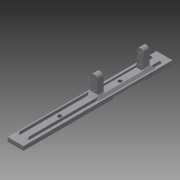
# Autodesk Inventor part: Top piece
Saved by Autodesk Inventor 2015 (Build 190159000, 159)
## iProperties
Created: 2014-11-22
Part Number: Top piece
Material: Generic
Document SubType Name: Modeling
Designer: jesse
Density: 1 g/cm^3
Appearance: Default
Author: jesse
Autodesk Inventor part; units mm, degrees
ref_plane "YZ Plane" through (0, 0, 0) normal (1, 0, 0) x (0, 1, 0)
ref_plane "XZ Plane" through (0, 0, 0) normal (0, 1, 0) x (-1, 0, 0)
ref_plane "XY Plane" through (0, 0, 0) normal (0, 0, 1) x (1, 0, 0)
sketch "Sketch1" plane through (0, 0, 0) normal (0, 0, 1) x (1, 0, 0)
  line L0 (10.1192, 6.6438) -> (35.5192, 6.6438)
  line L1 (35.5192, 6.6438) -> (35.5192, 0.2938)
  line L2 (35.5192, 0.2938) -> (10.1192, 0.2938)
  line L3 (10.1192, 0.2938) -> (10.1192, 6.6438)
  point P0 (0, 0)
  dimension "d0" = 25.4
  dimension "d1" = 6.35
  constraints: 8 end point, 2 parallel, 1 horizontal, 1 perpendicular
  measures "d0" distance of L1.end L2.end
  measures "d1" distance of L0.end L1.end
extrude "Extrusion1" add sketch "Sketch1" along normal blind 237.8075
sketch "Sketch2" plane through (10.1192, 6.6438, 0) normal (0, 1, 0) x (1, 0, 0)
  line L0 (0, 0) -> (25.4, 0) projected
  line L1 (0, 0) -> (0, -237.8075) projected
  line L2 (25.4, -237.8075) -> (0, -237.8075) projected
  line L3 (25.4, 0) -> (25.4, -237.8075) projected
  line L4 (12.7, 0) -> (12.7, -237.8075) construction
  line L5 (25.4, -237.8075) -> (0, -237.8075) construction
  line L6 (0, 0) -> (0, -237.8075) construction
  line L7 (0, -167.1637) -> (25.4, -167.1637) construction
  line L8 (0, -70.6437) -> (25.4, -70.6437) construction
  line L9 (25.4, 0) -> (25.4, -237.8075) construction
  circle A0 centre (12.7, -70.6437) radius 3.175
  circle A1 centre (12.7, -167.1637) radius 3.175
  line L10 (32.1721, -167.1637) -> (32.1721, -237.8075) construction
  line L11 (29.604, -70.6437) -> (29.604, 0) construction
  point P0 (-10.1192, 0)
  dimension "d6" = 6.35
  dimension "d7" = 6.35
  dimension "d10" = 96.52
  constraints: 10 end point, 8 point on line, 4 midpoint, 2 centre point, 2 parallel, 2 perpendicular, 1 vertical
  measures "d6" diameter of A0
  measures "d7" diameter of A1
  measures "d10" distance between parallel lines of L7 L8
extrude "Extrusion2" cut sketch "Sketch2" against normal through all contours A0 | A1
sketch "Sketch3" plane through (10.1192, 0.2938, 0) normal (-1, 0, 0) x (0, 0, 1)
  line L0 (44.8421, -2.7964) -> (94.9957, -2.7964)
  line L1 (94.9957, -2.7964) -> (94.9957, 2.2087)
  line L2 (94.9957, 2.2087) -> (44.8421, 2.2087)
  line L3 (44.8421, 2.2087) -> (44.8421, -2.7964)
  point P0 (0, -0.2938)
  constraints: 8 end point, 2 parallel, 1 horizontal, 1 perpendicular
extrude "Extrusion3" cut sketch "Sketch3" against normal through all
sketch "Sketch4" plane through (10.1192, 6.6438, 0) normal (0, 1, 0) x (1, 0, 0)
  line L0 (18.35, -38.735) -> (6.35, -38.735) projected
  line L1 (6.35, -102.735) -> (18.35, -102.735) projected
  line L2 (18.35, -38.735) -> (7.105, -38.735)
  line L3 (7.105, -38.735) -> (7.105, -29.21)
  line L4 (7.105, -29.21) -> (18.35, -29.21)
  line L5 (18.35, -29.21) -> (18.35, -38.735)
  line L6 (18.35, -102.735) -> (6.35, -102.735)
  line L7 (6.35, -102.735) -> (6.35, -112.26)
  line L8 (6.35, -112.26) -> (18.35, -112.26)
  line L9 (18.35, -112.26) -> (18.35, -102.735)
  point P0 (-10.1192, 0)
  dimension "d13" = 9.525
  dimension "d14" = 9.525
  constraints: 16 end point, 4 parallel, 2 horizontal, 2 perpendicular
  measures "d13" distance of L2.end L3.end
  measures "d14" distance of L7.end L6.end
extrude "Extrusion4" add sketch "Sketch4" along normal blind 30.1625
chamfer "Chamfer1" distance 4.7625 angle 45 2 edges at (22.8467, 6.6438, 29.21) (22.4692, 6.6438, 112.26)
sketch "Sketch5" plane through (16.4692, 36.8063, 112.26) normal (0, 0, 1) x (1, 0, 0)
  circle A0 centre (6, -22.1625) radius 1.3525 projected
  circle A1 centre (6, -6.1625) radius 1.3525 projected
  point P0 (-16.4692, -36.8063)
extrude "Extrusion5" cut sketch "Sketch5" against normal through all
fillet "Fillet1" radius 6.35 4 edges at (16.4692, 36.8063, 107.4975) (28.4692, 36.8063, 107.4975) (17.2242, 36.8063, 33.9725) (28.4692, 36.8063, 33.9725)
chamfer "Chamfer2" distance 4.7625 angle 45 4 edges at (16.4692, 6.6438, 109.8788) (28.4692, 6.6438, 109.8788) (28.4692, 6.6438, 31.5913) (17.2242, 6.6438, 31.5913)
sketch "Sketch6" plane through (10.1192, 6.6438, 0) normal (0, 1, 0) x (1, 0, 0)
  line L0 (25.4, -237.8075) -> (0, -237.8075) projected
  line L1 (18.6927, -237.8075) -> (21.1555, -237.8075)
  line L2 (21.1555, -212.4075) -> (21.1555, -112.0518)
  line L3 (21.1555, -112.0518) -> (18.6927, -112.0518)
  line L4 (18.6927, -112.0518) -> (18.6927, -212.4075)
  line L5 (6.7073, -237.8075) -> (4.2445, -237.8075)
  line L6 (4.2445, -212.4075) -> (4.2445, -112.0518)
  line L7 (4.2445, -112.0518) -> (6.7073, -112.0518)
  line L8 (6.7073, -112.0518) -> (6.7073, -212.4075)
  line L9 (25.4, 0) -> (25.4, -237.8075) projected
  line L10 (0, 0) -> (0, -237.8075) projected
  line L11 (21.1555, -171.8415) -> (25.4, -171.8415)
  line L12 (4.2445, -171.8415) -> (0, -171.8415)
  line L13 (20.8665, -0.289) -> (18.4037, -0.289)
  line L14 (18.4037, -34.2615) -> (20.8665, -34.2615)
  line L15 (7.105, -29.21) -> (2.3425, -24.4475) projected
  line L16 (3.9555, -0.289) -> (6.4182, -0.289)
  line L17 (6.4182, -28.5232) -> (3.9555, -28.5232)
  line L18 (31.115, -212.4075) -> (-5.715, -212.4075) projected
  point P0 (-10.1192, 0)
  point P1 (21.1555, -225.1075)
  point P2 (18.6927, -225.1075)
  point P3 (6.7073, -225.1075)
  point P4 (4.2445, -225.1075)
  constraints: 28 end point, 13 point on line, 6 parallel, 5 horizontal, 3 perpendicular, 2 collinear
extrude "Extrusion6" add sketch "Sketch6" along normal blind 4.7625 draft -20 contours L18 L4 L3 L2 | L18 L6 L7 L8
sketch "Sketch7" plane through (10.1192, 6.6438, 0) normal (0, 1, 0) x (1, 0, 0)
  line L0 (18.35, -90.5879) -> (18.35, -50.8821) construction
  line L1 (6.35, -50.8821) -> (6.35, -90.5879) construction
  line L2 (18.35, -99.735) -> (18.35, -41.735) construction
  line L3 (6.35, -99.735) -> (18.35, -99.735) construction
  line L4 (6.35, -41.735) -> (6.35, -99.735) construction
  line L5 (18.35, -41.735) -> (6.35, -41.735) construction
  circle A0 centre (12.35, -54.735) radius 1.3525 construction
  circle A1 centre (12.35, -62.735) radius 1.3525 construction
  circle A2 centre (12.35, -78.735) radius 1.3525 construction
  circle A3 centre (12.35, -86.735) radius 1.3525 construction
  line L6 (1.5875, -102.735) -> (23.1125, -102.735) projected
  line L7 (23.1125, -38.735) -> (2.3425, -38.735) projected
  line L8 (25.4, 0) -> (25.4, -44.8421) projected
  line L9 (18.35, -102.735) -> (25.4, -102.735)
  line L10 (25.4, -102.735) -> (25.4, -38.735)
  line L11 (25.4, -38.735) -> (18.35, -38.735)
  line L12 (18.35, -38.735) -> (18.35, -102.735)
  line L13 (0, 0) -> (0, -237.8075) projected
  line L14 (0, -102.735) -> (6.35, -102.735)
  line L15 (6.35, -102.735) -> (6.35, -38.735)
  line L16 (6.35, -38.735) -> (0, -38.735)
  line L17 (0, -38.735) -> (0, -102.735)
  point P0 (-10.1192, 0)
  constraints: 16 end point, 5 point on line, 4 parallel, 2 horizontal, 2 perpendicular
extrude "Extrusion7" add sketch "Sketch7" along normal blind 3.175 contours L14 L13 L16 L7 L15 L6 | L12 L7 L11 L8 L10 L9 L6
sketch "Sketch8" plane through (35.5192, 6.6438, 38.735) normal (0, 0, -1) x (-1, 0, 0)
  line L0 (5.4625, 3.175) -> (2.2875, 0) projected
  line L1 (0, 3.175) -> (5.4625, 3.175) projected
  line L2 (0, 0) -> (0, 3.175) projected
  line L3 (2.2875, 0) -> (0, 0) projected
  line L4 (23.0575, 0) -> (19.8825, 3.175) projected
  line L5 (25.4, 0) -> (23.0575, 0) projected
  line L6 (25.4, 0) -> (25.4, 3.175) projected
  line L7 (19.8825, 3.175) -> (25.4, 3.175) projected
  point P0 (35.5192, -6.6438)
extrude "Extrusion8" cut sketch "Sketch8" against normal through all
body "Solid1"
